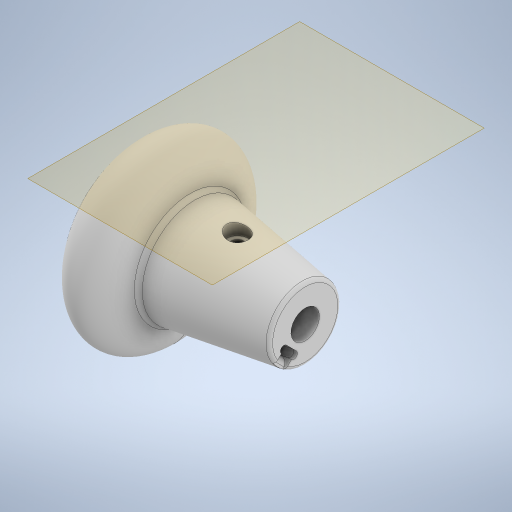
# Autodesk Inventor part: Joystick V1
Saved by Autodesk Inventor 2024.2 (Build 282272000, 272)
## iProperties
Created: 2024-06-04
Part Number: Joystick V1
Material: Generic
Document SubType Name: Modeling
Designer: ljubopudar
Density: 1 g/cm^3
Appearance: Default
Author: ljubopudar
Autodesk Inventor part; units mm, degrees
ref_plane "YZ Plane" through (0, 0, 0) normal (1, 0, 0) x (0, 1, 0)
ref_plane "XZ Plane" through (0, 0, 0) normal (0, 1, 0) x (-1, 0, 0)
sketch "Sketch1" plane through (0, 0, 0) normal (0, 1, 0) x (-1, 0, 0)
  line L0 (0, 0) -> (0, -9.1423)
  line L1 (0, 0) -> (32, 0)
  line L2 (30.8967, -14.7626) -> (0.8477, -10.1307)
  line L3 (32, 0) -> (50, 0)
  line L4 (50, 0) -> (40.8153, 0)
  line L5 (50, 0) -> (49, 0)
  arc A0 (0, -9.1423) -> (0.8477, -10.1307) centre (1, -9.1423) ccw
  line L6 (0, 0) -> (50, 0)
  arc A1 (32.2601, -15.636) -> (30.8967, -14.7626) centre (30.592, -16.7393) ccw
  ellipse E0 centre (40.8153, 0) end of major axis (40.6749, 24.9129) minor radius 11.0798 (32.2601, -15.636) -> (51.8953, 0) ccw
  line L7 (48.1114, 0) -> (58.1415, 0)
  point P0 (0, -10)
  point P1 (40.0027, -25)
  point P2 (0, -4.5712)
  point P3 (41, 0)
  dimension "d56" = 11.0798
  dimension "d0" = 10
  dimension "d11" = 1
  dimension "d19" = 25
  dimension "d20" = 2
  dimension "d34" = 16.7393
  dimension "d55" = 30.592
  dimension "d58" = 41
  dimension "d59" = 11.08
  constraints: 16 end point, 8 point on line, 4 point on circle, 3 tangent, 2 centre point, 2 midpoint, 1 coincident, 1 collinear, 1 horizontal, 1 vertical, 4 other
  measures "d0" distance of L0.start point (0, -10)
  measures "d11" radius of A0
  measures "d19" vertical distance of L4.end point (40.003, -25)
  measures "d20" radius of A1
  measures "d34" distance from line of L1 A1.centre
  measures "d55" distance from line of L0 A1.centre
  measures "d58" distance of point (41, 0) L0.start
  measures "d59" distance of point (51.895, 0) L4.end
revolve "Revolution1" add sketch "Sketch1" angle 360 about axis through (0, 0, 0) along (-1, 0, 0)
sketch "Sketch2" plane through (0, 0, 0) normal (1, 0, 0) x (0, 0, -1)
  circle A0 centre (0, 0) radius 3.5
  dimension "d23" = 7
  constraints: 1 centre point, 1 coincident
  measures "d23" diameter of A0
extrude "Extrusion1" cut sketch "Sketch2" against normal blind 33
sketch "Sketch3" plane through (0, 0, 0) normal (1, 0, 0) x (0, 0, -1)
  line L0 (-3.1336, 0) -> (-3.6885, 0)
  line L1 (-3.6885, 0) -> (-3.6885, 0.2927)
  line L2 (-3.6885, 0.2927) -> (-3.1336, 0.2927)
  line L3 (-3.1336, 0.2927) -> (-3.1336, 0)
  point P0 (0, 0)
  constraints: 8 end point, 2 parallel, 1 horizontal, 1 perpendicular
extrude "Extrusion2" cut sketch "Sketch3" against normal blind 1
ref_plane "Work Plane2" through (0, 0, 0) normal (0, 0, 1) x (1, 0, 0)
ref_plane "Work Plane1" through (0, 0, 3.5) normal (0, 0, 1) x (1, 0, 0)
sketch "Sketch4" plane through (-33, 0, 0) normal (1, 0, 0) x (0, 0, -1)
  point P0 (0, 0)
sketch "Sketch5" plane through (-33, 0, 0) normal (1, 0, 0) x (0, 0, -1)
  circle A0 centre (0, 0) radius 3.5 projected
extrude "Extrusion3" add sketch "Sketch5" along normal blind 1
sketch "Sketch6" plane through (0, 0, 0) normal (0, 0, 1) x (1, 0, 0)
  arc A0 (-50, 0) -> (-50.007, -0.7117) centre (-13.7112, -0.7117) ccw projected
  line L0 (-32, 3.5) -> (-32, -3.5) projected
  line L1 (-50, 0) -> (-47, 0)
  line L2 (-47, 0) -> (-47, 14.6)
  line L3 (-47, 14.6) -> (-34, 14.6)
  arc A1 (-32.4002, 15.8847) -> (-38.4604, 24.3486) centre (-58.7032, 3.4532) ccw projected
  line L4 (-34, 14.6) -> (-34, 0)
  line L5 (-34, 0) -> (-47, 0)
  line L6 (-57.4495, 0) -> (-57.4495, 24.5134)
  line L7 (-57.4495, 24.5134) -> (-47, 25.0676)
  line L8 (-47, 25.0676) -> (-47, 14.6)
  line L9 (-57.4495, 0) -> (-50, 0)
  line L10 (0, 9.1423) -> (0, -9.1423) projected
  point P0 (0, 0)
  dimension "d60" = 2
  dimension "d61" = 14.6
  dimension "d62" = 13
  dimension "d63" = 34
  constraints: 18 end point, 3 perpendicular, 3 vertical, 2 horizontal, 1 parallel, 1 point on line
  measures "d60" distance between parallel lines of L0 L4
  measures "d61" distance between parallel lines of L5 L3
  measures "d62" distance between parallel lines of L2 L4
  measures "d63" distance between parallel lines of L10 L4
revolve "Revolution2" cut sketch "Sketch6" angle 360 about axis through (-34, 0, 0) along (-1, 0, 0)
sketch "Sketch9" plane through (-34, 0, 0) normal (-1, 0, 0) x (0, 0, 1)
  line L0 (0, 0) -> (-33.4008, 0)
  line L1 (-33.4008, 0) -> (0, 0)
  line L2 (0, 0) -> (0, 44.3398)
  circle A0 centre (0, 0) radius 20.711 projected
  line L3 (0, 44.3398) -> (0, 0)
  line L4 (0, 0) -> (-26.5133, 21.5799)
  constraints: 10 end point, 2 collinear, 1 horizontal, 1 vertical
sketch "Sketch11" plane through (-34, 0, 0) normal (-1, 0, 0) x (0, 0, 1)
  point P0 (0, 0)
sketch "Sketch12" plane through (-34, 0, 0) normal (-1, 0, 0) x (0, 0, 1)
  point P0 (0, 0)
sketch "Sketch13" plane through (-47, 0, 0) normal (-1, 0, 0) x (0, 0, 1)
  point P0 (0, 0)
sketch "Sketch14" plane through (-47, 0, 0) normal (-1, 0, 0) x (0, 0, 1)
  arc A0 (3.4877, 0.2927) -> (3.5, 0) centre (0, 0) ccw projected
  arc A1 (-10.7168, -2.8277) -> (-6.9787, -8.6106) centre (0, 0) ccw construction
  circle A2 centre (0, 0) radius 11 construction
  arc A3 (-6.9261, -8.5457) -> (0, -11) centre (0, 0) ccw construction
  circle A4 centre (0, 0) radius 14.6 projected
  line L0 (-14.6, 0) -> (-11.6, 0)
  line L1 (-11.6, 0) -> (-10.6, 0)
  line L2 (-10.6, 0) -> (-10.6, -2)
  line L3 (-10.6, -2) -> (-12.6, -2)
  line L4 (-12.6, -2) -> (-12.6, 2)
  line L5 (-12.6, 2) -> (-10.6, 2)
  line L6 (-10.6, 2) -> (-10.6, 0)
  dimension "d65" = 22
  dimension "d67" = 3
  dimension "d68" = 1
  dimension "d69" = 2
  dimension "d70" = 2
  dimension "d71" = 4
  constraints: 14 end point, 5 perpendicular, 4 point on circle, 3 coincident, 2 centre point, 2 point on line, 1 horizontal, 1 horizontal alignment, 1 vertical alignment, 3 other
  measures "d67" distance of L0.start L0.end
  measures "d68" distance of L0.end L1.end
  measures "d69" distance of L1.end L2.end
  measures "d70" distance of L2.end L3.end
  measures "d71" distance of L3.end L4.end
extrude "Extrusion7" cut sketch "Sketch14" against normal blind 15 contours L4 L5 L6 L1 L0 | L0 L1 L2 L3 L4
sketch "Sketch17" plane through (-34, 0, 0) normal (-1, 0, 0) x (0, 0, 1)
  circle A0 centre (0, 0) radius 3.5 projected
  circle A1 centre (0, 0) radius 12 construction
  line L0 (-4.243, -12) -> (-11.3461, -4.9865)
  line L1 (-4.243, -12) -> (-11.3461, -4.9865) construction
  line L2 (-3.3647, -11.1105) -> (-10.4678, -4.097)
  line L3 (-12.2243, -5.8759) -> (-5.1213, -12.8895)
  arc A2 (-5.1213, -12.8895) -> (-3.3647, -11.1105) centre (-4.243, -12) ccw
  arc A3 (-10.4678, -4.097) -> (-12.2243, -5.8759) centre (-11.3461, -4.9865) ccw
  point P0 (0, 0)
  point P1 (-7.7945, -8.4932)
  dimension "d74" = 24
  dimension "d76" = 2.5
  constraints: 10 end point, 4 point on circle, 4 tangent, 3 centre point, 1 coincident, 1 midpoint, 1 parallel
  measures "d74" diameter of A1
  measures "d76" diameter of A3
sketch "Sketch18" plane through (0, 0, 0) normal (1, 0, 0) x (0, 0, -1)
  line L0 (3.3647, -11.1105) -> (10.4678, -4.097) projected
  line L1 (12.2243, -5.8759) -> (5.1213, -12.8895) projected
  arc A0 (12.2243, -5.8759) -> (10.4678, -4.097) centre (11.3461, -4.9865) ccw projected
  arc A1 (3.3647, -11.1105) -> (5.1213, -12.8895) centre (4.243, -12) ccw projected
  line L2 (5.9163, -3.1567) -> (3.07, -5.9672) construction
  line L3 (5.2137, -2.4452) -> (2.3674, -5.2556)
  line L4 (3.7726, -6.6787) -> (6.6189, -3.8683)
  arc A2 (6.6189, -3.8683) -> (5.2137, -2.4452) centre (5.9163, -3.1567) ccw
  arc A3 (2.3674, -5.2556) -> (3.7726, -6.6787) centre (3.07, -5.9672) ccw
  line L5 (0, 0) -> (7.7578, -7.8766)
  point P0 (4.4932, -4.562)
  dimension "d77" = 4
  dimension "d78" = 2
  constraints: 10 end point, 4 point on circle, 4 tangent, 2 centre point, 2 parallel, 1 midpoint, 1 point on line
  measures "d77" distance of L2.start L2.end
  measures "d78" diameter of A3
extrude "Extrusion8" cut sketch "Sketch17" against normal blind 1 contours A2 L3 A3 L2
extrude "Extrusion9" cut sketch "Sketch18" against normal blind 1 contours A2 L4 L5 L3 | L5 L4 A3 L3
loft "Loft2" cut section 1 edges at (-1, -6.6698, -2.3584) (-1, -5.2735, -5.1958) (-1, -2.4541, -6.6279) (-1, -3.8504, -3.7906) section 2 edges at (-33, -4.1082, -12.2355) (-33, -9.3827, -8.6728) (-33, -12.8783, -3.3535) (-33, -7.6038, -6.9163)
sketch "Sketch19" plane through (-33, -5.8759, -12.2243) normal (-0.1654073, 0.7017754, 0.6929298) x (0.9831269, 0.0616798, 0.1722122)
  line L0 (33.5323, 0.0781) -> (33.8492, -3.9093) projected
  line L1 (33.5323, 0.0781) -> (32.5492, 0) projected
  line L2 (32.5492, 0) -> (32.866, -3.9874) projected
  line L3 (33.8492, -3.9093) -> (32.866, -3.9874) projected
  point P0 (34.9108, -1.8106)
extrude "Extrusion10" cut sketch "Sketch19" against normal blind 3
fillet "Fillet1" radius 2 1 edges at (-1, -5.2735, -5.1958)
sketch "Sketch20" plane through (-47, -0.0022, 0.0149) normal (-1, 0, 0) x (0, 0, 1)
  circle A0 centre (-0.0149, 0.0022) radius 14.6 projected
  line L0 (-14.6149, 0.0022) -> (-16.6149, 0.0022)
  line L1 (-15.6508, 0.0022) -> (-24.9279, 0.0022) projected
  line L2 (-16.6149, 0.0022) -> (-19.1149, 0.0022)
  line L3 (-16.6149, 0.0022) -> (-16.6149, -2.4978)
  line L4 (-16.6149, -2.4978) -> (-25.2615, -2.4978)
  line L5 (-25.2615, -2.4978) -> (-25.2615, 2.3946)
  line L6 (-16.6149, 0.0022) -> (-16.6149, 2.5022)
  line L7 (-16.6149, 2.5022) -> (-20.9383, 2.5022)
  line L8 (-20.9383, 2.5022) -> (-25.2615, 2.5022)
  line L9 (-25.2615, 2.5022) -> (-25.2615, 2.3946)
  point P0 (-0.0149, 0.0022)
  point P1 (-20.8264, 0.0022)
  dimension "d90" = 2
  dimension "d91" = 2.5
  dimension "d92" = 2.5
  dimension "d93" = 2.5
  constraints: 18 end point, 3 perpendicular, 2 point on line, 2 vertical, 1 collinear, 1 horizontal, 1 horizontal alignment, 1 other
  measures "d90" distance of L0.start L0.end
  measures "d91" distance of L0.end L2.end
  measures "d92" distance of L0.end L3.end
  measures "d93" distance of L0.end L6.end
extrude "Extrusion11" cut sketch "Sketch20" against normal blind 1.5 contours L3 L4 L5 L9 L8 L7 L6
sketch "Sketch21" plane through (0, -5.2556, -2.3674) normal (1, 0, 0) x (0, 0.7026079, -0.7115772)
  circle A0 centre (2.008, 5.4031) radius 4
  dimension "d96" = 8
  constraints: 1 centre point, 1 coincident
  measures "d96" diameter of A0
extrude "Extrusion12" cut sketch "Sketch21" against normal up to surface (32 mm away)
ref_plane "Work Plane3" through (-40.928, 0, 24.913) normal (0, 0, 1) x (1, 0, 0)
sketch "Sketch22" plane through (-40.928, 0, 24.913) normal (0, 0, 1) x (1, 0, 0)
  line L0 (40.928, 4) -> (40.928, -4) projected
  line L1 (40.928, -4) -> (8.928, -4) projected
  line L2 (40.928, 4) -> (8.928, 4) projected
  line L3 (40.0804, 10.1307) -> (10.0313, 14.7626) projected
  line L4 (40.0804, -10.1307) -> (10.0313, -14.7626) projected
  line L5 (40.928, 9.1423) -> (40.928, -9.1423) projected
  line L6 (40.0804, 10.1307) -> (40.0804, -10.1307) projected
  line L7 (8.928, 4) -> (8.928, -4) projected
  circle A0 centre (21.928, 0) radius 1.5
  point P0 (40.928, 0)
  point P1 (40.928, -7.7575)
  point P2 (40.928, -4.9496)
  dimension "d99" = 3
  dimension "d103" = 19
  constraints: 1 centre point, 1 other
  measures "d99" diameter of A0
  measures "d103" distance from line of L0 A0.centre
extrude "Extrusion13" cut sketch "Sketch22" against normal blind 22 contours A0
sketch "Sketch23" plane through (-40.928, 0, 24.913) normal (0, 0, 1) x (1, 0, 0)
  circle A0 centre (21.9548, 0) radius 1.75
  point P0 (40.928, 0)
  dimension "d104" = 3.5
  constraints: 1 centre point, 1 other
  measures "d104" diameter of A0
extrude "Extrusion14" cut sketch "Sketch23" against normal blind 20
sketch "Sketch24" plane through (-40.928, 0, 24.913) normal (0, 0, 1) x (1, 0, 0)
  circle A0 centre (21.928, 0) radius 1.5 projected
  circle A1 centre (21.928, 0) radius 3
  point P0 (40.928, 0)
  dimension "d107" = 6
  constraints: 1 centre point, 1 coincident
  measures "d107" diameter of A1
extrude "Extrusion15" cut sketch "Sketch24" against normal blind 15
body "Solid1"
